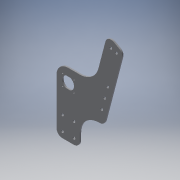
# Autodesk Inventor part: pG188Mount
Saved by Autodesk Inventor 2018 (Build 220112000, 112)
## iProperties
Created: 2017-02-20
Part Number: pG188Mount
Material: Generic
Document SubType Name: Sheet Metal
Designer: kingb
Density: 1 g/cm^3
Sheet Metal Rule: Default
Appearance: Default
Author: kingb
Autodesk Inventor part; units mm, degrees
ref_plane "YZ Plane" through (0, 0, 0) normal (1, 0, 0) x (0, 1, 0)
ref_plane "XZ Plane" through (0, 0, 0) normal (0, 1, 0) x (-1, 0, 0)
ref_plane "XY Plane" through (0, 0, 0) normal (0, 0, 1) x (1, 0, 0)
sketch "Sketch1" plane through (0, 0, 0) normal (0, 0, 1) x (1, 0, 0)
  line L0 (0, 0) -> (50.8, 0)
  line L1 (50.8, 0) -> (50.8, 27.1979)
  line L2 (50.8, 139.7) -> (0, 139.7)
  line L3 (0, 139.7) -> (0, 0)
  line L4 (128.6063, 161.9886) -> (104.1161, 68.3618)
  line L5 (418.4795, 73.9788) -> (-1.9313, 310.0684)
  arc A0 (104.1161, 68.3618) -> (50.8, 27.1979) centre (93.3487, 27.1979) ccw
  line L6 (128.6063, 161.9886) -> (145.6601, 227.1856)
  line L7 (63.1831, 62.4318) -> (91.6427, 171.2335) construction
  arc A1 (50.8, 139.7) -> (91.6427, 171.2335) centre (50.8, 181.9168) ccw
  line L8 (95.8188, 187.1988) -> (111.3222, 246.4687)
  line L9 (91.6427, 171.2335) -> (95.8188, 187.1988)
  line L10 (50.8, 27.1979) -> (50.8, 139.7) construction
  dimension "d0" = 50.8
  dimension "d1" = 139.7
  measures "d0" distance of L2.end L2.start
  measures "d1" distance of L2.start L0.end
extrude "Plate1" add sketch "Sketch1" along normal blind 3.048
fillet "Corner Round1" radius 25.4 1 edges at (50.8, 139.7, 1.524)
fillet "Corner Round1" radius 25.4 1 edges at (0, 139.7, 1.524)
fillet "Corner Round2" radius 12.7 2 edges at (50.8, 0, 1.524) (0, 0, 1.524)
sketch "Sketch2" plane through (0, 0, 0) normal (0, 0, -1) x (-1, 0, 0)
  arc A0 (-20.4, 99.125) -> (-20.4, 123.125) centre (-25.4, 111.125) ccw projected
  line L0 (-20.4, 123.125) -> (-30.4, 123.125) projected
  line L1 (-30.4, 99.125) -> (-20.4, 99.125) projected
  arc A1 (-30.4, 123.125) -> (-30.4, 99.125) centre (-25.4, 111.125) ccw projected
  circle A2 centre (-13.0256, 98.7506) radius 1.65 projected
  circle A3 centre (-37.7744, 123.4994) radius 1.65 projected
  circle A4 centre (-13.0256, 123.4994) radius 1.65 projected
  circle A5 centre (-37.7744, 98.7506) radius 1.65 projected
  point P0 (0, 0)
extrude "Extrusion1" cut sketch "Sketch2" against normal up to surface (3.048 mm away)
sketch "Sketch3" plane through (0, 0, 3.048) normal (0, 0, 1) x (1, 0, 0)
  circle A0 centre (38.1, 44.45) radius 2.9337 projected
  circle A1 centre (12.7, 44.45) radius 2.9337 projected
  circle A2 centre (12.7, 12.7) radius 2.9337 projected
  circle A3 centre (38.1, 12.7) radius 2.9337 projected
  circle A4 centre (12.7, 12.7) radius 2.9337 projected
  point P0 (0, 0)
extrude "Extrusion2" cut sketch "Sketch3" against normal up to surface (3.048 mm away)
fillet "Corner Round3" radius 12.7 1 edges at (104.1161, 68.3618, 1.524)
fillet "Corner Round3" radius 12.7 2 edges at (145.6601, 227.1856, 1.524) (111.3222, 246.4687, 1.524)
sketch "Sketch4" plane through (0, 0, 3.048) normal (0, 0, 1) x (1, 0, 0)
  line L0 (91.6427, 171.2335) -> (107.1596, 230.5549) projected
  line L1 (125.6647, 238.4145) -> (137.1107, 231.9868) projected
  line L2 (143.1788, 217.6995) -> (106.9555, 79.2171) projected
  line L3 (143.0742, 217.2996) -> (106.2143, 226.9411) construction
  line L4 (133.8968, 219.7001) -> (137.1107, 231.9868) construction
  circle A0 centre (118.501, 223.7273) radius 2.9337
  circle A1 centre (130.7876, 220.5134) radius 2.9337
  line L5 (143.0742, 217.2996) -> (130.7876, 220.5134) construction
  line L6 (106.2143, 226.9411) -> (118.501, 223.7273) construction
  line L7 (130.7876, 220.5134) -> (91.3386, 69.6992)
  arc A2 (94.3654, 69.7345) -> (50.8, 27.1979) centre (93.3487, 27.1979) ccw projected
  circle A3 centre (124.3599, 195.9402) radius 2.9337
  circle A4 centre (117.9322, 171.3669) radius 2.9337
  circle A5 centre (111.5045, 146.7937) radius 2.9337
  circle A6 centre (105.0768, 122.2204) radius 2.9337
  circle A7 centre (98.6491, 97.6472) radius 2.9337
  point P0 (0, 0)
  dimension "d13" = 12.7
  dimension "d14" = 5.8674
  dimension "d15" = 5.8674
  dimension "d16" = 12.7
  dimension "d17" = 12.7
  dimension "d21" = 25.4
  constraints: 10 end point, 7 centre point, 5 point on line, 2 perpendicular, 1 parallel, 1 point on circle, 11 other
  measures "d13" distance of L1.end L4.start
  measures "d14" diameter of A0
  measures "d15" diameter of A1
  measures "d16" distance of L3.start L5.end
  measures "d17" distance of L3.end L6.end
  measures "d21" distance of L5.end A3.centre
extrude "Extrusion3" cut sketch "Sketch4" against normal up to next contours A0 | A1 | A5 L7 | L7 A5 | A6 L7 | L7 A6 | A7 L7 | L7 A7
equation "\"d10\" = Thickness"
equation "\"BendRadius\" = Thickness"
equation "\"BendReliefWidth\" = Thickness"
equation "\"BendReliefDepth\" = 0.5 * Thickness"
equation "\"CornerReliefSize\" = 4 * Thickness"
equation "\"MinimumRemnant\" = 2 * Thickness"
equation "\"TransitionRadius\" = BendRadius"
equation "\"JacobiRadiusSize\" = Thickness"
equation "\"GapSize\" = Thickness"
equation "\"d2\" = BendRadius"
equation "\"Thickness\" = 3.048"
body "Solid1"
